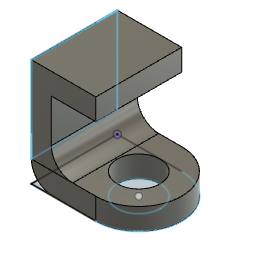
Assignment_03 (Autodesk Fusion 360 design; units mm, degrees)
Autodesk Fusion 360 part; units mm, degrees
sketch "Sketch1" plane through (0, 0, 0) normal (0, 1, 0) x (1, 0, 0)
  line L0 (0, 0) -> (30, 0)
  line L1 (30, -40) -> (0, -40)
  line L2 (0, -40) -> (0, 0)
  circle A0 centre (30, -20) radius 10
  arc A1 (30, -40) -> (30, 0) centre (30, -20) ccw
  dimension "d1" = 30
  dimension "d2" = 40
  dimension "d3" = 20
  constraint horizontal L0
  constraint horizontal L1
  constraint vertical L2
  constraint coincident L0.start L2.end
  constraint concentric A0 A1
  measures "d1" distance of L0.start L0.end
  measures "d2" distance of L0.start L1.end
  measures "d3" diameter of A0
sketch "Sketch2" plane through (0, 0, 0) normal (0, 0, 1) x (1, 0, 0)
  line L0 (10, 0) -> (9.2942, 0)
  line L1 (9.2942, 20) -> (9.2942, 40.06)
  line L2 (9.2942, 50.06) -> (0, 50.06)
  line L3 (0, 50.06) -> (0, 10)
  line L4 (50, 0) -> (9.2942, 0)
  line L5 (19.2942, 10) -> (50, 10)
  line L6 (50, 10) -> (50, 0)
  line L7 (0, 50.06) -> (30, 50.06)
  line L8 (30, 50.06) -> (30, 40.06)
  line L9 (30, 40.06) -> (9.2942, 40.06)
  line L10 (0, 40.06) -> (0, 50.06)
  arc A0 (0, 10) -> (10, 0) centre (10, 10) ccw
  arc A1 (9.2942, 20) -> (19.2942, 10) centre (19.2942, 20) ccw
  dimension "d4" = 50.06
  dimension "d5" = 10
  dimension "d6" = 30
  dimension "d7" = 10
  dimension "d8" = 10
  dimension "d9" = 10
  constraint horizontal L0
  constraint vertical L1
  constraint horizontal L2
  constraint vertical L3
  constraint horizontal L4
  constraint horizontal L5
  constraint vertical L6
  constraint horizontal L7
  constraint vertical L8
  constraint horizontal L9
  constraint vertical L10
  constraint coincident origin L0
  constraint coincident origin L3
  constraint tangent L0 A0
  constraint tangent L3 A0
  constraint coincident L0.end L1
  constraint tangent L5 A1
  constraint tangent L1 A1
  measures "d4" distance of origin L2.end
  measures "d5" distance of L4.start L5.end
  measures "d6" distance of L2.end L7.end
  measures "d7" distance of L2.end L10.start
  measures "d8" radius of A0
  measures "d9" radius of A1
sketch "Sketch3" plane through (0, 0, 0) normal (0, 0, 1) x (1, 0, 0)
sketch "Sketch4" plane through (0, 0, 0) normal (1, 0, 0) x (0, 0, -1)
  line L0 (-40, 10) -> (-40, 50)
  line L1 (-40, 50) -> (0, 50)
  line L2 (0, 50) -> (0, 10)
  line L3 (0, 10) -> (-40, 10)
  line L4 (-40, 10) -> (-40, 50)
  line L5 (-40, 50) -> (0, 50)
  line L6 (0, 50) -> (0, 10)
  constraint vertical L0
  constraint horizontal L1
  constraint vertical L2
  constraint horizontal L3
  constraint vertical L4
  constraint horizontal L5
  constraint vertical L6
extrude "Extrude1" add sketch "Sketch2" along normal blind 40 makes body 1
extrude "Extrude2" add sketch "Sketch1" along normal blind 10 separate body makes body 2
fillet "Fillet1" radius 10 1 edges at (0, 0, 20) on bodies 2
fillet "Fillet2" radius 20 1 edges at (50, 5, 0) on bodies 1
fillet "Fillet3" radius 20 1 edges at (50, 5, 40) on bodies 1
cylinder "CylinderPrimitive1" cut diameter 20 height 25 placed x (1, 0, 0) y (0, 0, -1) z (0, 1, 0) at (30, 0, 20) bodies 1
